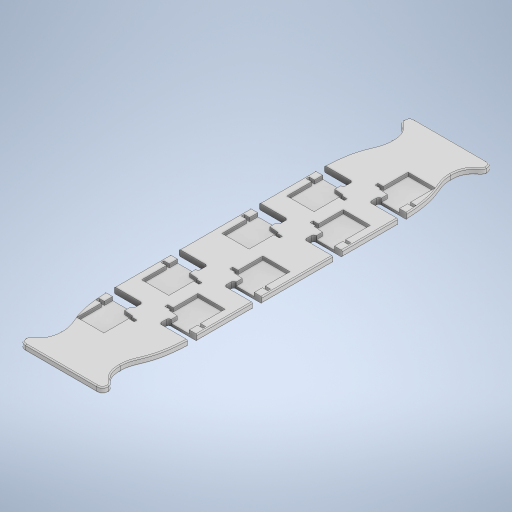
# Autodesk Inventor part: flipper_robot_v2_hull
Saved by Autodesk Inventor 2023.1 (Build 271208000, 208)
## iProperties
Created: 2025-10-23
Part Number: flipper_robot_v2_hull
Material: Generic
Document SubType Name: Modeling
Designer: Lars
Density: 1 g/cm^3
Appearance: Default
Author: Lars
Autodesk Inventor part; units mm, degrees
ref_plane "YZ Plane" through (0, 0, 0) normal (1, 0, 0) x (0, 1, 0)
ref_plane "XZ Plane" through (0, 0, 0) normal (0, 1, 0) x (-1, 0, 0)
ref_plane "XY Plane" through (0, 0, 0) normal (0, 0, 1) x (1, 0, 0)
sketch "Baseplate Profile" plane through (0, 0, 0) normal (0, 1, 0) x (-1, 0, 0)
  line L0 (-35, 125) -> (35, 125) construction
  line L1 (35, 125) -> (35, -125)
  line L2 (35, -125) -> (-35, -125) construction
  line L3 (-35, -125) -> (-35, 125)
  line L4 (-35, 125) -> (35, -125) construction
  line L5 (35, 125) -> (-35, -125) construction
  line L6 (25, -125) -> (25, -155) construction
  line L7 (35, -85) -> (35, -125) construction
  line L8 (35, -125) -> (25, -125) construction
  line L9 (25, -125) -> (25, -140) construction
  spline S0 degree 3 poles (35, -85) (35, -125) (25, -125) (25, -140) knots 1 1 1 1 2 2 2 2
  line L10 (25, -140) -> (25, -155) construction
  line L11 (25, -155) -> (35, -155) construction
  line L12 (35, -155) -> (35, -160) construction
  spline S1 degree 3 poles (25, -140) (25, -155) (35, -155) (35, -160) knots 1 1 1 1 2 2 2 2
  line L13 (35, -165) -> (35, -160) construction
  line L14 (35, -160) -> (35, -165) construction
  line L15 (35, -165) -> (30, -165) construction
  spline S2 degree 2 poles (35, -160) (35, -165) (30, -165) knots 1 1 1 2 2 2
  line L16 (30, -165) -> (0, -165)
  line L17 (0, -125) -> (0, -165) construction
  line L18 (-35, -85) -> (-35, -125) construction
  line L19 (-35, -125) -> (-25, -125) construction
  line L20 (-25, -125) -> (-25, -140) construction
  spline S3 degree 3 poles (-35, -85) (-35, -125) (-25, -125) (-25, -140) knots 1 1 1 1 2 2 2 2
  line L21 (-25, -140) -> (-25, -155) construction
  line L22 (-25, -155) -> (-35, -155) construction
  line L23 (-35, -155) -> (-35, -160) construction
  spline S4 degree 3 poles (-25, -140) (-25, -155) (-35, -155) (-35, -160) knots 1 1 1 1 2 2 2 2
  line L24 (-35, -160) -> (-35, -165) construction
  line L25 (-35, -165) -> (-30, -165) construction
  spline S5 degree 2 poles (-35, -160) (-35, -165) (-30, -165) knots 1 1 1 2 2 2
  line L26 (-30, -165) -> (0, -165)
  line L27 (35, 0) -> (-35, 0) construction
  line L28 (35, 85) -> (35, 125) construction
  line L29 (35, 125) -> (25, 125) construction
  line L30 (25, 125) -> (25, 140) construction
  spline S6 degree 3 poles (35, 85) (35, 125) (25, 125) (25, 140) knots 1 1 1 1 2 2 2 2
  line L31 (25, 140) -> (25, 155) construction
  line L32 (25, 155) -> (35, 155) construction
  line L33 (35, 155) -> (35, 160) construction
  spline S7 degree 3 poles (25, 140) (25, 155) (35, 155) (35, 160) knots 1 1 1 1 2 2 2 2
  line L34 (35, 160) -> (35, 165) construction
  line L35 (35, 165) -> (30, 165) construction
  spline S8 degree 2 poles (35, 160) (35, 165) (30, 165) knots 1 1 1 2 2 2
  line L36 (30, 165) -> (0, 165)
  spline S9 degree 3 poles (-35, 85) (-35, 125) (-25, 125) (-25, 140) knots 1 1 1 1 2 2 2 2
  line L37 (-35, 85) -> (-35, 125) construction
  line L38 (-35, 125) -> (-25, 125) construction
  line L39 (-25, 125) -> (-25, 140) construction
  spline S10 degree 3 poles (-25, 140) (-25, 155) (-35, 155) (-35, 160) knots 1 1 1 1 2 2 2 2
  line L40 (-25, 140) -> (-25, 155) construction
  line L41 (-25, 155) -> (-35, 155) construction
  line L42 (-35, 155) -> (-35, 160) construction
  spline S11 degree 2 poles (-35, 160) (-35, 165) (-30, 165) knots 1 1 1 2 2 2
  line L43 (-35, 160) -> (-35, 165) construction
  line L44 (-35, 165) -> (-30, 165) construction
  line L45 (-30, 165) -> (0, 165)
  point P0 (0, 0)
  point P1 (0, 0)
  point P2 (35, 85.0002)
  point P3 (-35, 85.0002)
  point P4 (-35, -85.0002)
  dimension "d8" = 70
  dimension "d9" = 250
  dimension "d97" = 30
  dimension "d99" = 40
  dimension "d110" = 5
  dimension "d111" = 5
  dimension "d112" = 25
  dimension "d113" = 35
  dimension "d114" = 10
  dimension "d115" = 10
  dimension "d116" = 5
  constraints: 28 end point, 28 symmetric about line, 6 midpoint, 5 coincident, 4 collinear, 3 perpendicular, 2 horizontal, 2 parallel, 2 point on line, 2 vertical, 36 other
  measures "d8" distance of L1.end L2.end
  measures "d9" distance of L0.end L1.end
  measures "d97" distance of L6.start L6.end
  measures "d99" distance of L7.start L7.end
  measures "d110" distance of L13.start L12.end
  measures "d111" distance of L14.end L15.end
  measures "d112" vertical distance of L9.end L15.end
  measures "d113" horizontal distance of L16.end L12.end
  measures "d114" distance of L7.end L8.end
  measures "d115" distance of L10.end L11.end
  measures "d116" distance of L11.end L12.end
extrude "Baseplate" add sketch "Baseplate Profile" along normal blind 5
sketch "Servo Feature Layout" plane through (0, 5, 0) normal (0, 1, 0) x (1, 0, 0)
  line L0 (-35, 85) -> (-35, -85.0002) construction
  line L1 (-35, -34) -> (35, -34) construction
  line L2 (35, -85.0002) -> (35, 85.0002) construction
  line L3 (35, -89) -> (35, -89) construction
  line L4 (-35, 34) -> (35, 34) construction
  line L5 (-35, 89) -> (35, 89) construction
  line L6 (-35, -93) -> (-11, -93)
  line L7 (-11, -93) -> (-11, -85)
  line L8 (-11, -85) -> (-35, -85)
  line L9 (-23, -93) -> (-23, -122.8) construction
  line L10 (-28.45, -93) -> (-28.45, -100)
  line L11 (-28.45, -100) -> (-33, -100)
  line L12 (-33, -100) -> (-33, -102.4)
  line L13 (-33, -102.4) -> (-28.45, -102.4)
  line L14 (-28.45, -102.4) -> (-28.45, -123.4)
  line L15 (-28.45, -123.4) -> (-5.45, -123.4)
  line L16 (-5.45, -123.4) -> (-5.45, -102.4)
  line L17 (-5.45, -102.4) -> (-0.9, -102.4)
  line L18 (-0.9, -102.4) -> (-0.9, -99.96)
  line L19 (-0.9, -99.96) -> (-5.45, -99.96)
  line L20 (-5.45, -99.96) -> (-5.45, -98.86)
  line L21 (-28.45, -93) -> (-13.15, -93)
  line L22 (-13.15, -93) -> (-13.15, -98.2)
  line L23 (-13.15, -98.2) -> (-5.45, -98.86)
  line L24 (-35, -38) -> (-11, -38)
  line L25 (-11, -38) -> (-11, -30)
  line L26 (-11, -30) -> (-35, -30)
  line L27 (-35, -30) -> (-35, -38)
  line L28 (-23, -38) -> (-23, -67.8) construction
  line L29 (-28.45, -38) -> (-28.45, -45)
  line L30 (-28.45, -45) -> (-33, -45)
  line L31 (-33, -45) -> (-33, -47.4)
  line L32 (-33, -47.4) -> (-28.45, -47.4)
  line L33 (-28.45, -47.4) -> (-28.45, -68.4)
  line L34 (-28.45, -68.4) -> (-5.45, -68.4)
  line L35 (-5.45, -68.4) -> (-5.45, -47.4)
  line L36 (-5.45, -47.4) -> (-0.9, -47.4)
  line L37 (-0.9, -47.4) -> (-0.9, -44.96)
  line L38 (-0.9, -44.96) -> (-5.45, -44.96)
  line L39 (-5.45, -44.96) -> (-5.45, -43.86)
  line L40 (-28.45, -38) -> (-13.15, -38)
  line L41 (-13.15, -38) -> (-13.15, -43.2)
  line L42 (-13.15, -43.2) -> (-5.45, -43.86)
  line L43 (-35, 34) -> (35, 34) construction
  line L44 (-35, 30) -> (-11, 30)
  line L45 (-11, 38) -> (-35, 38)
  line L46 (-11, 30) -> (-11, 38)
  line L47 (-35, 38) -> (-35, 30)
  line L48 (-28.45, 30) -> (-13.15, 30)
  line L49 (-13.15, 30) -> (-13.15, 24.8)
  line L50 (-28.45, 30) -> (-28.45, 23)
  line L51 (-28.45, 23) -> (-33, 23)
  line L52 (-33, 23) -> (-33, 20.6)
  line L53 (-33, 20.6) -> (-28.45, 20.6)
  line L54 (-28.45, -0.4) -> (-5.45, -0.4)
  line L55 (-28.45, 20.6) -> (-28.45, -0.4)
  line L56 (-23, 30) -> (-23, 0.2) construction
  line L57 (-5.45, 20.6) -> (-0.9, 20.6)
  line L58 (-0.9, 23.04) -> (-5.45, 23.04)
  line L59 (-0.9, 20.6) -> (-0.9, 23.04)
  line L60 (-5.45, 23.04) -> (-5.45, 24.14)
  line L61 (-13.15, 24.8) -> (-5.45, 24.14)
  line L62 (-5.45, -0.4) -> (-5.45, 20.6)
  line L63 (-35, 89) -> (35, 89) construction
  line L64 (-35, 85) -> (-11, 85)
  line L65 (-11, 93) -> (-35, 93)
  line L66 (-11, 85) -> (-11, 93)
  line L67 (-35, 93) -> (-35, 85)
  line L68 (-28.45, 85) -> (-13.15, 85)
  line L69 (-13.15, 85) -> (-13.15, 79.8)
  line L70 (-28.45, 85) -> (-28.45, 78)
  line L71 (-28.45, 78) -> (-33, 78)
  line L72 (-33, 78) -> (-33, 75.6)
  line L73 (-33, 75.6) -> (-28.45, 75.6)
  line L74 (-28.45, 54.6) -> (-5.45, 54.6)
  line L75 (-28.45, 75.6) -> (-28.45, 54.6)
  line L76 (-23, 85) -> (-23, 55.2) construction
  line L77 (-5.45, 75.6) -> (-0.9, 75.6)
  line L78 (-0.9, 78.04) -> (-5.45, 78.04)
  line L79 (-0.9, 75.6) -> (-0.9, 78.04)
  line L80 (-5.45, 78.04) -> (-5.45, 79.14)
  line L81 (-13.15, 79.8) -> (-5.45, 79.14)
  line L82 (-5.45, 54.6) -> (-5.45, 75.6)
  line L83 (35, 21) -> (35, 21) construction
  line L84 (35, -93) -> (35, -85)
  line L85 (35, -85) -> (11, -85)
  line L86 (11, -85) -> (11, -93)
  line L87 (11, -93) -> (35, -93)
  line L88 (33, -78) -> (33, -75.6)
  line L89 (33, -75.6) -> (28.45, -75.6)
  line L90 (28.45, -78) -> (33, -78)
  line L91 (28.45, -85) -> (28.45, -78)
  line L92 (23, -85) -> (23, -55.2) construction
  line L93 (28.45, -75.6) -> (28.45, -54.6)
  line L94 (28.45, -54.6) -> (5.45, -54.6)
  line L95 (5.45, -54.6) -> (5.45, -75.6)
  line L96 (5.45, -75.6) -> (0.9, -75.6)
  line L97 (0.9, -75.6) -> (0.9, -78.04)
  line L98 (0.9, -78.04) -> (5.45, -78.04)
  line L99 (5.45, -78.04) -> (5.45, -79.14)
  line L100 (13.15, -79.8) -> (5.45, -79.14)
  line L101 (13.15, -85) -> (13.15, -79.8)
  line L102 (28.45, -85) -> (13.15, -85)
  line L103 (-35, -89) -> (35, -89) construction
  line L104 (-35, -93) -> (-35, -85)
  line L105 (35, -34) -> (35, -34) construction
  line L106 (33, -20.6) -> (28.45, -20.6)
  line L107 (33, -23) -> (33, -20.6)
  line L108 (28.45, -23) -> (33, -23)
  line L109 (35, -30) -> (11, -30)
  line L110 (11, -38) -> (35, -38)
  line L111 (35, -38) -> (35, -30)
  line L112 (0.9, -20.6) -> (0.9, -23.04)
  line L113 (5.45, -20.6) -> (0.9, -20.6)
  line L114 (0.9, -23.04) -> (5.45, -23.04)
  line L115 (11, -30) -> (11, -38)
  line L116 (28.45, -30) -> (13.15, -30)
  line L117 (28.45, -30) -> (28.45, -23)
  line L118 (13.15, -30) -> (13.15, -24.8)
  line L119 (13.15, -24.8) -> (5.45, -24.14)
  line L120 (5.45, -23.04) -> (5.45, -24.14)
  line L121 (23, -30) -> (23, -0.2) construction
  line L122 (28.45, -20.6) -> (28.45, 0.4)
  line L123 (5.45, 0.4) -> (5.45, -20.6)
  line L124 (28.45, 0.4) -> (5.45, 0.4)
  line L125 (35, 34) -> (35, 34) construction
  line L126 (33, 47.4) -> (28.45, 47.4)
  line L127 (33, 45) -> (33, 47.4)
  line L128 (28.45, 45) -> (33, 45)
  line L129 (35, 38) -> (11, 38)
  line L130 (11, 30) -> (35, 30)
  line L131 (35, 30) -> (35, 38)
  line L132 (0.9, 47.4) -> (0.9, 44.96)
  line L133 (5.45, 47.4) -> (0.9, 47.4)
  line L134 (0.9, 44.96) -> (5.45, 44.96)
  line L135 (11, 38) -> (11, 30)
  line L136 (28.45, 38) -> (13.15, 38)
  line L137 (28.45, 38) -> (28.45, 45)
  line L138 (13.15, 38) -> (13.15, 43.2)
  line L139 (13.15, 43.2) -> (5.45, 43.86)
  line L140 (5.45, 44.96) -> (5.45, 43.86)
  line L141 (23, 38) -> (23, 67.8) construction
  line L142 (28.45, 47.4) -> (28.45, 68.4)
  line L143 (5.45, 68.4) -> (5.45, 47.4)
  line L144 (28.45, 68.4) -> (5.45, 68.4)
  line L145 (35, 89) -> (35, 89) construction
  line L146 (33, 102.4) -> (28.45, 102.4)
  line L147 (33, 100) -> (33, 102.4)
  line L148 (28.45, 100) -> (33, 100)
  line L149 (35, 93) -> (11, 93)
  line L150 (11, 85) -> (35, 85)
  line L151 (35, 85) -> (35, 93)
  line L152 (0.9, 102.4) -> (0.9, 99.96)
  line L153 (5.45, 102.4) -> (0.9, 102.4)
  line L154 (0.9, 99.96) -> (5.45, 99.96)
  line L155 (11, 93) -> (11, 85)
  line L156 (28.45, 93) -> (13.15, 93)
  line L157 (28.45, 93) -> (28.45, 100)
  line L158 (13.15, 93) -> (13.15, 98.2)
  line L159 (13.15, 98.2) -> (5.45, 98.86)
  line L160 (5.45, 99.96) -> (5.45, 98.86)
  line L161 (23, 93) -> (23, 122.8) construction
  line L162 (28.45, 102.4) -> (28.45, 123.4)
  line L163 (5.45, 123.4) -> (5.45, 102.4)
  line L164 (28.45, 123.4) -> (5.45, 123.4)
  point P0 (0, 0)
  point P1 (-35, 125)
  point P2 (-35, -125)
  point P3 (35, -125)
  point P4 (35, 125)
  point P5 (-35, -34)
  point P6 (-35, 34)
  point P7 (-35, 89)
  point P8 (35, 57)
  dimension "d18" = 34
  dimension "d19" = 55
  dimension "d20" = 34
  dimension "d21" = 55
  dimension "d23" = 8
  dimension "d24" = 29.8
  dimension "d25" = 7
  dimension "d26" = 4.55
  dimension "d27" = 2.4
  dimension "d28" = 21
  dimension "d30" = 10
  dimension "d31" = 23
  dimension "d38" = 4.55
  dimension "d39" = 4.55
  dimension "d40" = 1.1
  dimension "d41" = 2.44
  dimension "d42" = 15.3
  dimension "d43" = 5.2
  dimension "d44" = 94.899
  dimension "d46" = 8
  dimension "d47" = 29.8
  dimension "d48" = 7
  dimension "d49" = 4.55
  dimension "d50" = 2.4
  dimension "d51" = 21
  dimension "d52" = 10
  dimension "d53" = 23
  dimension "d54" = 4.55
  dimension "d55" = 4.55
  dimension "d56" = 1.1
  dimension "d57" = 2.44
  dimension "d58" = 15.3
  dimension "d59" = 5.2
  dimension "d60" = 94.899
  dimension "d61" = 8
  dimension "d62" = 29.8
  dimension "d63" = 7
  dimension "d64" = 4.55
  dimension "d65" = 2.4
  dimension "d66" = 21
  dimension "d67" = 10
  dimension "d68" = 23
  dimension "d69" = 4.55
  dimension "d70" = 4.55
  dimension "d71" = 1.1
  dimension "d72" = 2.44
  dimension "d73" = 15.3
  dimension "d74" = 5.2
  dimension "d75" = 94.899
  dimension "d76" = 8
  dimension "d77" = 29.8
  dimension "d78" = 7
  dimension "d79" = 4.55
  dimension "d80" = 2.4
  dimension "d81" = 21
  dimension "d82" = 10
  dimension "d83" = 23
  dimension "d84" = 4.55
  dimension "d85" = 4.55
  dimension "d86" = 1.1
  dimension "d87" = 2.44
  dimension "d88" = 15.3
  dimension "d89" = 5.2
  dimension "d90" = 94.899
  constraints: 326 end point, 40 point on line, 27 perpendicular, 24 horizontal, 12 vertical, 8 midpoint, 7 parallel, 3 symmetric about line, 1 collinear
  measures "d18" distance from line of L1 point (0, 0)
  measures "d19" distance between parallel lines of L3 L1
  measures "d20" distance from line of L4 point (0, 0)
  measures "d21" distance between parallel lines of L5 L4
  measures "d23" distance of L7.end L6.end
  measures "d24" distance of L9.start L9.end
  measures "d25" distance of L10.start L10.end
  measures "d26" distance of L10.end L11.end
  measures "d27" distance of L11.end L12.end
  measures "d28" distance of L13.end L14.end
  measures "d30" distance between parallel lines of L12 L9
  measures "d31" distance of L14.end L15.end
  measures "d38" distance between parallel lines of L16 L18
  measures "d39" distance of L18.end L19.end
  measures "d40" distance of L19.end L20.end
  measures "d41" distance between parallel lines of L19 L17
  measures "d42" distance of L10.start L21.end
  measures "d43" distance of L21.end L22.end
  measures "d44" angle of L22 L23
  measures "d46" distance of L26.start L24.end
  measures "d47" distance of L28.start L28.end
  measures "d48" distance of L40.start L29.end
  measures "d49" distance of L29.end L30.end
  measures "d50" distance of L30.end L31.end
  measures "d51" distance of L32.end L34.start
  measures "d52" distance between parallel lines of L31 L28
  measures "d53" distance of L34.start L34.end
  measures "d54" distance between parallel lines of L35 L37
  measures "d55" distance of L38.start L38.end
  measures "d56" distance of L38.end L39.end
  measures "d57" distance between parallel lines of L38 L36
  measures "d58" distance of L40.start L40.end
  measures "d59" distance of L40.end L41.end
  measures "d60" angle of L41 L42
  measures "d61" distance of L46.end L44.end
  measures "d62" distance of L56.start L56.end
  measures "d63" distance of L48.start L51.start
  measures "d64" distance of L51.start L51.end
  measures "d65" distance of L51.end L52.end
  measures "d66" distance of L53.end L54.start
  measures "d67" distance between parallel lines of L52 L56
  measures "d68" distance of L54.start L54.end
  measures "d69" distance between parallel lines of L62 L59
  measures "d70" distance of L59.end L60.start
  measures "d71" distance of L60.start L60.end
  measures "d72" distance between parallel lines of L58 L57
  measures "d73" distance of L48.start L48.end
  measures "d74" distance of L48.end L49.end
  measures "d75" angle of L49 L61
  measures "d76" distance of L66.end L64.end
  measures "d77" distance of L76.start L76.end
  measures "d78" distance of L68.start L71.start
  measures "d79" distance of L71.start L71.end
  measures "d80" distance of L71.end L72.end
  measures "d81" distance of L73.end L74.start
  measures "d82" distance between parallel lines of L72 L76
  measures "d83" distance of L74.start L74.end
  measures "d84" distance between parallel lines of L82 L79
  measures "d85" distance of L79.end L80.start
  measures "d86" distance of L80.start L80.end
  measures "d87" distance between parallel lines of L78 L77
  measures "d88" distance of L68.start L68.end
  measures "d89" distance of L68.end L69.end
  measures "d90" angle of L69 L81
extrude "Horn Clearance Slot" cut sketch "Servo Feature Layout" against normal blind 5 contours L104 L8 L7 L6 | L27 L26 L25 L24 | L47 L45 L46 L44 | L67 L65 L66 L64 | L87 L86 L85 L84 | L109 L111 L110 L115 | L129 L131 L130 L135 | L149 L151 L150 L155
extrude "Servo Mount Pockets" cut sketch "Servo Feature Layout" against normal blind 3 contours L6 L22 L23 L20 L19 L18 L17 L16 L15 L14 L13 L12 L11 L10 | L24 L41 L42 L39 L38 L37 L36 L35 L34 L33 L32 L31 L30 L29 | L44 L49 L61 L60 L58 L59 L57 L62 L54 L55 L53 L52 L51 L50 | L64 L69 L81 L80 L78 L79 L77 L82 L74 L75 L73 L72 L71 L70 | L85 L101 L100 L99 L98 L97 L96 L95 L94 L93 L89 L88 L90 L91 | L107 L108 L117 L109 L118 L119 L120 L114 L112 L113 L123 L124 L122 L106 | L127 L128 L137 L129 L138 L139 L140 L134 L132 L133 L143 L144 L142 L126 | L147 L148 L157 L149 L158 L159 L160 L154 L152 L153 L163 L164 L162 L146
fillet "Fillets (Baseplate)" radius 0.9 40 edges at (30, 5, -153.75) (33.75, 5, -163.75) (0, 5, -165) (-33.75, 5, -163.75) (-30, 5, -153.75) (-29.4637, 5, -123.3068) (29.4637, 5, -123.3068) (-30, 0, -153.75) (-29.4637, 0, -123.3068) (0, 0, -165) (33.75, 0, -163.75) (30, 0, -153.75) (29.4637, 0, -123.3068) (-33.75, 0, -163.75) (-35, 5, -61.5) (-35, 0, -61.5) (-35, 0, 0) (-35, 5, 0) (-35, 5, 61.5) (-35, 0, 61.5) (-30, 0, 153.75) (-33.75, 0, 163.75) (0, 0, 165) (33.75, 0, 163.75) (30, 0, 153.75) (29.4637, 0, 123.3068) (-29.4637, 0, 123.3068) (-30, 5, 153.75) (-33.75, 5, 163.75) (0, 5, 165) (33.75, 5, 163.75) (30, 5, 153.75) (29.4637, 5, 123.3068) (-29.4637, 5, 123.3068) (35, 5, 61.5) (35, 5, 0) (35, 5, -61.5) (35, 0, -61.5) (35, 0, 0) (35, 0, 61.5)
fillet "Fillets (Clearance Slot)" radius 2 16 edges at (11, 2.5, 85) (11, 2.5, 93) (11, 2.5, 30) (11, 2.5, 38) (11, 2.5, -38) (11, 2.5, -30) (11, 2.5, -93) (11, 2.5, -85) (-11, 2.5, -93) (-11, 2.5, -85) (-11, 2.5, -38) (-11, 2.5, -30) (-11, 2.5, 30) (-11, 2.5, 38) (-11, 2.5, 85) (-11, 2.5, 93)
body "Solid1"
